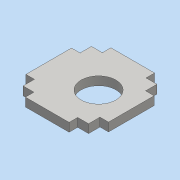
# Autodesk Inventor part: Camera-Holder_Bearing-Ring-Outer-Left
Saved by Autodesk Inventor 2016 SP1 (Build 200210100, 210)
## iProperties
Created: 2016-01-20
Part Number: Camera-Holder_Bearing-Ring-Outer-Left
Material: Generic
Document SubType Name: Modeling
Designer: Mohamed A.
Density: 1 g/cm^3
Appearance: Default
Author: Mohamed A.
Autodesk Inventor part; units mm, degrees
ref_plane "YZ Plane" through (0, 0, 0) normal (1, 0, 0) x (0, 1, 0)
ref_plane "XZ Plane" through (0, 0, 0) normal (0, 1, 0) x (-1, 0, 0)
ref_plane "XY Plane" through (0, 0, 0) normal (0, 0, 1) x (1, 0, 0)
sketch "Sketch1" plane through (0, 0, 0) normal (0, 0, 1) x (1, 0, 0)
  circle A0 centre (0, 0) radius 6.096
  line L0 (11.5, 8) -> (8.5, 8)
  line L1 (8.5, 8) -> (8.5, 12)
  line L2 (8.5, -12) -> (8.5, -8)
  line L3 (8.5, -8) -> (11.5, -8)
  line L4 (-10.6667, -15) -> (-10.6667, -12)
  line L5 (-10.6667, -12) -> (-14.5, -12)
  line L6 (4.6667, -15) -> (4.6667, -12)
  line L7 (4.6667, -12) -> (8.5, -12)
  line L8 (-17.5, -8) -> (-14.5, -8)
  line L9 (-14.5, -8) -> (-14.5, -12)
  line L10 (-17.5, 8) -> (-14.5, 8)
  line L11 (-14.5, 8) -> (-14.5, 12)
  line L12 (-10.6667, 15) -> (-10.6667, 12)
  line L13 (-10.6667, 12) -> (-14.5, 12)
  line L14 (8.5, 12) -> (4.6667, 12)
  line L15 (4.6667, 12) -> (4.6667, 15)
  line L16 (-10.6667, 15) -> (4.6667, 15)
  line L17 (-17.5, -8) -> (-17.5, 8)
  line L18 (4.6667, -15) -> (-10.6667, -15)
  line L19 (11.5, -8) -> (11.5, 8)
  line L20 (-20.9424, 0) -> (31.3224, 0) construction
  line L21 (0, 16.7256) -> (0, -15.9648) construction
  line L22 (4.6667, 12) -> (-10.6667, -12) construction
  line L23 (4.6667, -12) -> (-10.6667, 12) construction
  point P0 (-3, 0)
  dimension "d0" = 12.192
  dimension "d3" = 3
  dimension "d5" = 3
  dimension "d6" = 3
  dimension "d7" = 16
  dimension "d15" = 30
  dimension "d16" = 3
  dimension "d20" = 14.5
  dimension "d21" = 8.5
  dimension "d22" = 23
  dimension "d23" = 15.3333
  dimension "d24" = 24
  constraints: 48 end point, 12 point on line, 8 perpendicular, 4 horizontal, 3 collinear, 2 midpoint, 2 vertical, 1 centre point, 1 coincident, 1 parallel, 2 other
  measures "d0" diameter of A0
  measures "d3" distance of L0.start L0.end
  measures "d5" distance of L8.start L8.end
  measures "d6" distance of L12.start L12.end
  measures "d7" distance between parallel lines of L3 L0
  measures "d15" distance between parallel lines of L18 L16
  measures "d16" distance of L6.start L6.end
  measures "d20" distance between parallel lines of L21 L11
  measures "d21" distance between parallel lines of L21 L1
  measures "d22" distance between parallel lines of L11 L1
  measures "d23" distance between parallel lines of L12 L15
  measures "d24" distance between parallel lines of L7 L14
extrude "Extrusion1" add sketch "Sketch1" along normal blind 3
equation "\"d7\" = 0.666667 * d24"
equation "\"d23\" = 0.666667 * d22"
body "Solid1"
